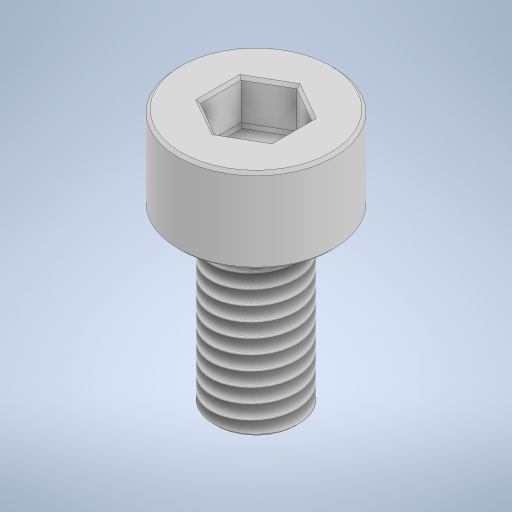
# Autodesk Inventor part: M3 X 6
Saved by Autodesk Inventor 2023 (Build 270158000, 158)
## iProperties
Created: 2023-04-10
Part Number: M3 X 6
Material: Generic
Document SubType Name: Modeling
Designer: Louis
Density: 1 g/cm^3
Appearance: Default
Author: Louis
Autodesk Inventor part; units mm, degrees
ref_plane "YZ Plane" through (0, 0, 0) normal (1, 0, 0) x (0, 1, 0)
ref_plane "XZ Plane" through (0, 0, 0) normal (0, 1, 0) x (-1, 0, 0)
ref_plane "XY Plane" through (0, 0, 0) normal (0, 0, 1) x (1, 0, 0)
sketch "Sketch1" plane through (0, 0, 0) normal (0, 0, 1) x (1, 0, 0)
  line L0 (0, 9) -> (2.75, 9)
  line L1 (2.75, 9) -> (2.75, 6)
  line L2 (2.75, 6) -> (1.5, 6)
  line L3 (1.5, 6) -> (1.5, 0)
  line L4 (1.5, 0) -> (0, 0)
  line L5 (0, 0) -> (0, 9)
  dimension "d0" = 2.75
  dimension "d1" = 3
  dimension "d2" = 6
  dimension "d3" = 1.5
  constraints: 12 end point, 5 perpendicular, 1 horizontal
  measures "d0" distance of L0.start L0.end
  measures "d1" distance of L0.end L1.end
  measures "d2" distance of L2.end L3.end
  measures "d3" distance of L3.end L4.end
revolve "Revolution1" add sketch "Sketch1" angle 360 about axis through (0, 0, 0) along (0, 1, 0)
thread "Thread1" size "M3x0.5" class "6g" standard "ANSI Metric M Profile" full length
sketch "Sketch3" plane through (0, 9, 0) normal (0, 1, 0) x (1, 0, 0)
  line L0 (1.25, -0.7217) -> (0, -1.4434)
  line L1 (0, -1.4434) -> (-1.25, -0.7217)
  line L2 (-1.25, -0.7217) -> (-1.25, 0.7217)
  line L3 (-1.25, 0.7217) -> (0, 1.4434)
  line L4 (0, 1.4434) -> (1.25, 0.7217)
  line L5 (1.25, 0.7217) -> (1.25, -0.7217)
  point P0 (0, 0)
  point P1 (0, 0)
  dimension "d13" = 2.5
  constraints: 12 end point, 1 coincident, 13 other
  measures "d13" distance between parallel lines of L5 L2
extrude "Extrusion2" cut sketch "Sketch3" against normal blind 1.5
chamfer "Chamfer2" distance 0.1 angle 45 16 edges at (0.625, 9, 1.0825) (1.25, 9, 0) (1.25, 7.5, 0) (0.625, 9, -1.0825) (0.625, 7.5, -1.0825) (-0.625, 9, -1.0825) (-0.625, 7.5, -1.0825) (-1.25, 7.5, 0) (-1.25, 9, 0) (-0.625, 7.5, 1.0825) (-0.625, 9, 1.0825) (0.625, 7.5, 1.0825) (-2.75, 9, 0) (-2.75, 6, 0) (-1.5, 6, 0) (-1.5, 0, 0)
body "Solid1"
